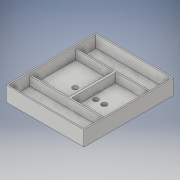
# Autodesk Inventor part: Base no cutouts.stl
Saved by Autodesk Inventor 2018 (Build 220112000, 112)
## iProperties
Created: 2018-02-19
Part Number: Base no cutouts.stl
Material: Generic
Document SubType Name: Modeling
Designer: Eric G
Density: 1 g/cm^3
Appearance: Default
Author: Eric G
Autodesk Inventor part; units mm, degrees
ref_plane "YZ Plane" through (0, 0, 0) normal (1, 0, 0) x (0, 1, 0)
ref_plane "XZ Plane" through (0, 0, 0) normal (0, 1, 0) x (-1, 0, 0)
ref_plane "XY Plane" through (0, 0, 0) normal (0, 0, 1) x (1, 0, 0)
sketch "Sketch2" plane through (0, 0, 0) normal (0, 1, 0) x (-1, 0, 0)
  line L0 (170.5606, 186.8878) -> (-160.1389, 186.8878)
  line L1 (-160.1389, 186.8878) -> (-160.1389, -194.6885)
  line L2 (-160.1389, -194.6885) -> (170.5606, -194.6885)
  line L3 (170.5606, -194.6885) -> (170.5606, 186.8878)
  constraints: 8 end point, 2 parallel, 1 horizontal, 1 perpendicular
extrude "Extrusion1" add sketch "Sketch2" along normal blind 12.7
sketch "Sketch4" plane through (0, 12.7, 0) normal (0, 1, 0) x (1, 0, 0)
  line L0 (-170.5606, -186.8878) -> (160.1389, -186.8878) projected
  line L1 (160.1389, -186.8878) -> (160.1389, 194.6885) projected
  line L2 (-170.5606, -186.8878) -> (160.1389, -186.8878)
  line L3 (160.1389, -186.8878) -> (160.1389, 194.6885)
  line L4 (160.1389, 194.6885) -> (-170.5606, 194.6885)
  line L5 (-170.5606, 194.6885) -> (-170.5606, -186.8878)
  point P0 (0, 0)
  constraints: 8 end point, 2 parallel, 1 horizontal, 1 perpendicular
extrude "Extrusion2" add sketch "Sketch4" along normal blind 50.8
sketch "Sketch5" plane through (0, 63.5, 0) normal (0, 1, 0) x (1, 0, 0)
  line L0 (-165.3089, -181.8398) -> (155.2723, -181.8398)
  line L1 (155.2723, -181.8398) -> (155.2723, 188.9245)
  line L2 (155.2723, 188.9245) -> (-165.3089, 188.9245)
  line L3 (-165.3089, 188.9245) -> (-165.3089, -181.8398)
  point P0 (0, 0)
  constraints: 8 end point, 2 parallel, 1 horizontal, 1 perpendicular
extrude "Extrusion3" cut sketch "Sketch5" against normal blind 50.8
sketch "Sketch9" plane through (0, 12.7, 0) normal (0, 1, 0) x (1, 0, 0)
  line L0 (-165.3089, -181.8398) -> (-165.3089, 188.9245) projected
  line L1 (155.2723, 188.9245) -> (155.2723, -181.8398) projected
  line L2 (-165.3089, 109.1943) -> (155.2723, 109.1943)
  line L3 (155.2723, 109.1943) -> (155.2723, 103.846)
  line L4 (155.2723, 103.846) -> (-165.3089, 103.846)
  line L5 (-165.3089, 103.846) -> (-165.3089, 109.1943)
  line L6 (-165.3089, -90.4753) -> (155.2723, -90.4753)
  line L7 (155.2723, -90.4753) -> (155.2723, -84.2356)
  line L8 (155.2723, -84.2356) -> (-165.3089, -84.2356)
  line L9 (-165.3089, -84.2356) -> (-165.3089, -90.4753)
  line L10 (-5.0183, 103.846) -> (4.0112, 103.846)
  line L11 (4.0112, 103.846) -> (4.0112, -84.2356)
  line L12 (4.0112, -84.2356) -> (-5.0183, -84.2356)
  line L13 (-5.0183, -84.2356) -> (-5.0183, 103.846)
  point P0 (0, 0)
  constraints: 24 end point, 6 parallel, 5 point on line, 3 horizontal, 3 perpendicular, 1 midpoint
extrude "Extrusion6" add sketch "Sketch9" along normal blind 38.1 contours L0 L8 L1 L6 | L0 L2 L1 L4 | L13 L4 L11 L8
sketch "Sketch16" plane through (0, 12.7, 0) normal (0, 1, 0) x (1, 0, 0)
  circle A0 centre (23.4848, 0) radius 10.6311
  circle A1 centre (-26.8974, 0) radius 10.5141
  circle A2 centre (59.1623, 0) radius 11.4331
  circle A3 centre (-64.229, 0) radius 10.9108
  point P0 (0, 0)
  constraints: 4 centre point
extrude "Extrusion10" cut sketch "Sketch16" against normal blind 25.4
body "Solid1"
